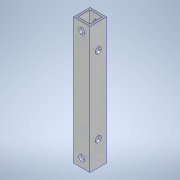
# Autodesk Inventor part: ハンド9x9_3
Saved by Autodesk Inventor 2020.3 (Build 243373000, 373)
## iProperties
Created: 2020-05-31
Part Number: ハンド9x9_3
Material: アルミニウム 6061
Document SubType Name: Modeling
Designer: totot
Density: 2.7 g/cm^3
Appearance: アルミニウム - フラット
Mass: 5.84359 g
Surface Area: 37.8156 cm^2
Volume: 2.16429 cm^3
Author: totot
Autodesk Inventor part; units mm, degrees
ref_plane "YZ Plane" through (0, 0, 0) normal (1, 0, 0) x (0, 1, 0)
ref_plane "XZ Plane" through (0, 0, 0) normal (0, 1, 0) x (-1, 0, 0)
ref_plane "XY Plane" through (0, 0, 0) normal (0, 0, 1) x (1, 0, 0)
sketch "スケッチ1" plane through (0, 0, 0) normal (0, 1, 0) x (-1, 0, 0)
  line L0 (0, 0) -> (-9, 0)
  line L1 (-9, 0) -> (-9, 9)
  line L2 (-9, 9) -> (0, 9)
  line L3 (0, 9) -> (0, 0)
  line L4 (-1.2, 7.8) -> (-7.8, 7.8)
  line L5 (-7.8, 7.8) -> (-7.8, 1.2)
  line L6 (-7.8, 1.2) -> (-1.2, 1.2)
  line L7 (-1.2, 1.2) -> (-1.2, 7.8)
  dimension "d0" = 9
  dimension "d1" = 9
  dimension "d2" = 1.2
  dimension "d3" = 1.2
  dimension "d4" = 1.2
  dimension "d5" = 1.2
  constraints: 16 end point, 4 parallel, 2 horizontal, 2 perpendicular
  measures "d0" distance of L1.end L2.end
  measures "d1" distance of L0.end L1.end
  measures "d2" distance between parallel lines of L2 L4
  measures "d3" distance between parallel lines of L0 L6
  measures "d4" distance between parallel lines of L7 L3
  measures "d5" distance between parallel lines of L1 L5
extrude "押し出し1" add sketch "スケッチ1" along normal blind 73.5
sketch "スケッチ2" plane through (0, 0, 9) normal (0, 0, 1) x (1, 0, 0)
  line L0 (0, 0) -> (0, 73.5) projected
  line L1 (0, 0) -> (9, 0) projected
  line L2 (0, 73.5) -> (9, 73.5) projected
  point P0 (4.5, 69)
  point P1 (4.5, 4.5)
  dimension "d8" = 4.5
  dimension "d9" = 4.5
  dimension "d10" = 4.5
  dimension "d11" = 4.5
  measures "d8" distance from line of L0 point (4.5, 69)
  measures "d9" distance from line of L0 point (4.5, 4.5)
  measures "d10" distance from line of L1 point (4.5, 4.5)
  measures "d11" distance from line of point (4.5, 69) L2
hole "穴1" at (4.5, 69, 9) at (4.5, 4.5, 9) direction (0, 0, -1) diameter 3.3 end through all
sketch "スケッチ3" plane through (9, 0, 9) normal (1, 0, 0) x (0, 0, -1)
  line L0 (0, 0) -> (0, 73.5) projected
  line L1 (0, 73.5) -> (9, 73.5) projected
  line L2 (0, 0) -> (9, 0) projected
  point P0 (4.5, 60)
  point P1 (4.5, 13.5)
  dimension "d19" = 4.5
  dimension "d20" = 4.5
  dimension "d21" = 13.5
  dimension "d22" = 13.5
  measures "d19" distance from line of L0 point (4.5, 60)
  measures "d20" distance from line of L0 point (4.5, 13.5)
  measures "d21" distance from line of point (4.5, 60) L1
  measures "d22" distance from line of point (4.5, 13.5) L2
hole "穴2" at (9, 60, 4.5) at (9, 13.5, 4.5) direction (-1, 0, 0) diameter 3.3 end through all
sketch "スケッチ4" plane through (9, 0, 0) normal (0, 0, -1) x (-1, 0, 0)
  line L0 (9, 0) -> (9, 73.5) projected
  line L1 (0, 73.5) -> (9, 73.5) projected
  line L2 (0, 0) -> (9, 0) projected
  point P0 (4.5, 48.5)
  point P1 (4.5, 25)
  dimension "d30" = 4.5
  dimension "d31" = 4.5
  dimension "d32" = 25
  dimension "d33" = 25
  measures "d30" distance from line of point (4.5, 48.5) L0
  measures "d31" distance from line of L0 point (4.5, 25)
  measures "d32" distance from line of point (4.5, 48.5) L1
  measures "d33" distance from line of point (4.5, 25) L2
hole "穴3" at (4.5, 48.5, 0) at (4.5, 25, 0) direction (0, 0, 1) diameter 4 end through all
equation "\"d3\" = d2"
equation "\"d4\" = d3"
equation "\"d5\" = d4"
equation "\"d9\" = d8"
equation "\"d10\" = d9"
equation "\"d11\" = d8"
equation "\"d20\" = d19"
equation "\"d22\" = d21"
equation "\"d33\" = d32"
